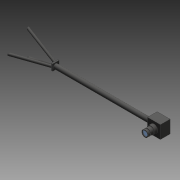
# Autodesk Inventor part: 摄像头
Saved by Autodesk Inventor 2016 (Build 200138000, 138)
## iProperties
Created: 2019-05-19
Part Number: 摄像头
Material: 橡胶
Document SubType Name: Modeling
Designer: oldboy
Density: 0.93 g/cm^3
Appearance: 橡胶 - 黑色
Author: oldboy
Autodesk Inventor part; units mm, degrees
ref_plane "YZ Plane" through (0, 0, 0) normal (1, 0, 0) x (0, 1, 0)
ref_plane "XZ Plane" through (0, 0, 0) normal (0, 1, 0) x (-1, 0, 0)
sketch "草图1" plane through (0, 0, 0) normal (0, 1, 0) x (-1, 0, 0)
  circle A0 centre (0, 0) radius 5
  dimension "d0" = 10
  constraints: 1 centre point, 1 coincident
  measures "d0" diameter of A0
extrude "拉伸1" add sketch "草图1" along normal blind 2
sketch "草图2" plane through (0, 2, 0) normal (0, 1, 0) x (1, 0, 0)
  circle A0 centre (0, 0) radius 5 projected
  circle A1 centre (0, 0) radius 4
  dimension "d3" = 8
  constraints: 1 centre point, 1 coincident
  measures "d3" diameter of A1
extrude "拉伸2" add sketch "草图2" along normal blind 1 contours A1
sketch "草图3" plane through (0, 3, 0) normal (0, 1, 0) x (1, 0, 0)
  circle A0 centre (0, 0) radius 5 projected
extrude "拉伸3" add sketch "草图3" along normal blind 5
sketch "草图4" plane through (0, 0, 0) normal (0, -1, 0) x (1, 0, 0)
  circle A0 centre (0, 0) radius 5 projected
  circle A1 centre (0, 0) radius 4 projected
extrude "拉伸4" add sketch "草图4" along normal blind 1
sketch "草图5" plane through (0, 8, 0) normal (0, 1, 0) x (1, 0, 0)
  circle A0 centre (0, 0) radius 6
  dimension "d10" = 12
  constraints: 1 centre point, 1 coincident
  measures "d10" diameter of A0
extrude "拉伸5" add sketch "草图5" along normal blind 5
sketch "草图6" plane through (0, 13, 0) normal (0, 1, 0) x (1, 0, 0)
  line L0 (-10, -10) -> (10, -10)
  line L1 (10, -10) -> (10, 10)
  line L2 (10, 10) -> (-10, 10)
  line L3 (-10, 10) -> (-10, -10)
  line L4 (-10, -10) -> (10, 10) construction
  line L5 (10, -10) -> (-10, 10) construction
  point P0 (0, 0)
  dimension "d13" = 20
  constraints: 12 end point, 2 midpoint, 2 parallel, 2 perpendicular, 1 horizontal
  measures "d13" distance of L1.end L2.end
extrude "拉伸6" add sketch "草图6" along normal blind 15
sketch "草图7" plane through (-10, 13, -10) normal (-1, 0, 0) x (0, 0, 1)
  line L0 (20, 0) -> (20, 15) construction
  line L1 (20, 0) -> (0, 0) construction
  line L2 (20, 15) -> (0, 0) construction
  line L3 (20, 0) -> (0, 15) construction
  circle A0 centre (10, 7.5) radius 3.5
  point P0 (10, -13)
  dimension "d16" = 7
  constraints: 4 end point, 1 centre point, 1 midpoint
  measures "d16" diameter of A0
extrude "拉伸7" add sketch "草图7" along normal blind 150
sketch "草图8" plane through (-160, 20.5, 0) normal (-1, 0, 0) x (0, 0, 1)
  line L0 (-4.7374, 5.2626) -> (5.2626, 5.2626)
  line L1 (5.2626, 5.2626) -> (5.2626, -4.7374)
  line L2 (5.2626, -4.7374) -> (-4.7374, -4.7374)
  line L3 (-4.7374, -4.7374) -> (-4.7374, 5.2626)
  line L4 (-4.7374, 5.2626) -> (5.2626, -4.7374) construction
  line L5 (5.2626, 5.2626) -> (-4.7374, -4.7374) construction
  point P0 (0, -20.5)
  point P1 (0.2626, 0.2626)
  dimension "d19" = 10
  constraints: 12 end point, 2 midpoint, 2 parallel, 2 perpendicular, 1 horizontal
  measures "d19" distance of L0.end L1.end
extrude "拉伸8" add sketch "草图8" along normal blind 2
sketch "草图9" plane through (-162, 20.5, 0) normal (-1, 0, 0) x (0, 0, 1)
  line L0 (0, 0) -> (0, 3) construction
  line L1 (0, 0) -> (-2.5981, -1.5) construction
  line L2 (0, 0) -> (2.5981, -1.5) construction
  line L3 (0, 0) -> (-4.7226, 0) construction
  circle A0 centre (-2.5981, 1.5) radius 2
  circle A1 centre (0, -3) radius 2
  circle A2 centre (2.5981, 1.5) radius 2
  point P0 (0, -20.5)
  dimension "d22" = 120
  dimension "d23" = 120
  dimension "d24" = 3
  dimension "d26" = 3
  dimension "d27" = 3
  constraints: 8 end point, 3 centre point, 1 horizontal, 1 vertical
  measures "d22" angle of L0 L1
  measures "d23" angle of L2 L1
  measures "d24" distance of L0.start L0.end
  measures "d26" distance of L0.start L1.end
  measures "d27" distance of L0.start L2.end
ref_plane "工作平面2" through (-212.499, 20.5, 0) normal (-1, 0, 0) x (0, 0, 1)
ref_plane "工作平面1" through (-161, 20.5, 0) normal (-1, 0, 0) x (0, 0, 1)
sketch "草图10" plane through (-212.499, 20.5, 0) normal (-1, 0, 0) x (0, 0, 1)
  line L0 (0, 18.3) -> (0, -29.3) construction
  line L1 (-30.8, -20.5) -> (30.8, -20.5) construction
  circle A0 centre (0, -20.5) radius 2
  circle A1 centre (-20, 9.5) radius 2
  circle A2 centre (20, 9.5) radius 2
  dimension "d32" = 4
  dimension "d33" = 4
  dimension "d34" = 30
  dimension "d35" = 20
  constraints: 3 centre point, 1 coincident, 1 symmetric about line, 1 other
  measures "d32" diameter of A0
  measures "d33" diameter of A1
  measures "d34" distance from line of L1 A1.centre
  measures "d35" distance from line of L0 A1.centre
loft "放样1" add profiles "草图10", "草图9" contours A0 / A1
loft "放样2" add profiles "草图9", "草图10" contours A2 / A2
loft "放样3" add profiles "草图9", "草图10" contours A0 / A1
